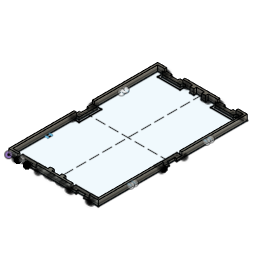
eNSPanel v2.1.4 enclosure (Autodesk Fusion 360 design; units mm, degrees)
Autodesk Fusion 360 part; units mm, degrees
note: some values were not read from the file. Chosen so that the rebuilt part matches the saved one: which bodies a step acts on; which face or edge a step refers to.
sketch "Sketch1" plane through (0, 0, 0) normal (0, 0, 1) x (1, 0, 0)
  line L0 (21, 0) -> (21, 3.8)
  line L1 (21, 3.8) -> (7, 3.8)
  line L2 (7, 3.8) -> (7, 0)
  line L3 (17, 0) -> (17, 1.4)
  line L4 (17, 1.4) -> (11, 1.4)
  line L5 (11, 1.4) -> (11, 0)
  line L6 (0, 57.2) -> (68.8, 57.2) construction
  line L7 (34.4, 114.4) -> (34.4, 0) construction
  line L8 (47.8, 0) -> (47.8, 3.8)
  line L9 (47.8, 3.8) -> (61.8, 3.8)
  line L10 (61.8, 3.8) -> (61.8, 0)
  line L11 (51.8, 1.4) -> (57.8, 1.4)
  line L12 (57.8, 1.4) -> (57.8, 0)
  line L13 (51.8, 0) -> (51.8, 1.4)
  line L14 (7, 110.6) -> (7, 114.4)
  line L15 (21, 110.6) -> (7, 110.6)
  line L16 (21, 114.4) -> (21, 110.6)
  line L17 (17, 113) -> (11, 113)
  line L18 (11, 113) -> (11, 114.4)
  line L19 (17, 114.4) -> (17, 113)
  line L20 (47.8, 114.4) -> (47.8, 110.6)
  line L21 (47.8, 110.6) -> (61.8, 110.6)
  line L22 (51.8, 113) -> (57.8, 113)
  line L23 (51.8, 114.4) -> (51.8, 113)
  line L24 (57.8, 113) -> (57.8, 114.4)
  line L25 (61.8, 110.6) -> (61.8, 114.4)
  line L26 (68.8, 54.2) -> (67.4, 54.2)
  line L27 (67.4, 54.2) -> (67.4, 60.2)
  line L28 (67.4, 60.2) -> (68.8, 60.2)
  line L29 (68.8, 50.2) -> (65, 50.2)
  line L30 (65, 50.2) -> (65, 64.2)
  line L31 (65, 64.2) -> (68.8, 64.2)
  line L32 (3.8, 64.2) -> (0, 64.2)
  line L33 (3.8, 50.2) -> (3.8, 64.2)
  line L34 (0, 50.2) -> (3.8, 50.2)
  line L35 (0, 54.2) -> (1.4, 54.2)
  line L36 (1.4, 54.2) -> (1.4, 60.2)
  line L37 (1.4, 60.2) -> (0, 60.2)
  line L38 (7, 0) -> (11, 0)
  line L39 (17, 0) -> (21, 0)
  line L40 (0, 0) -> (11, 0)
  line L41 (17, 0) -> (51.8, 0)
  line L42 (57.8, 0) -> (68.8, 0)
  line L43 (68.8, 0) -> (68.8, 54.2)
  line L44 (68.8, 60.2) -> (68.8, 114.4)
  line L45 (68.8, 64.2) -> (68.8, 60.2)
  line L46 (68.8, 54.2) -> (68.8, 50.2)
  line L47 (0, 114.4) -> (0, 60.2)
  line L48 (0, 54.2) -> (0, 0)
  line L49 (11, 114.4) -> (0, 114.4)
  line L50 (68.8, 114.4) -> (57.8, 114.4)
  line L51 (51.8, 114.4) -> (17, 114.4)
  line L52 (18.6, 1.6) -> (50.2, 1.6)
  line L53 (50.2, 1.6) -> (50.2, 3)
  line L54 (50.2, 3) -> (59.4, 3)
  line L55 (59.4, 3) -> (59.4, 1.6)
  line L56 (59.4, 1.6) -> (67.2, 1.6)
  line L57 (67.2, 1.6) -> (67.2, 52.6)
  line L58 (67.2, 52.6) -> (65.8, 52.6)
  line L59 (65.8, 52.6) -> (65.8, 61.8)
  line L60 (65.8, 61.8) -> (67.2, 61.8)
  line L61 (67.2, 61.8) -> (67.2, 112.8)
  line L62 (67.2, 112.8) -> (59.4, 112.8)
  line L63 (18.6, 1.6) -> (18.6, 3)
  line L64 (18.6, 3) -> (9.4, 3)
  line L65 (9.4, 3) -> (9.4, 1.6)
  line L66 (8.5, 1.6) -> (9.4, 1.6)
  line L67 (1.6, 52.6) -> (1.6, 1.6)
  line L68 (1.6, 1.6) -> (9.4, 1.6)
  line L69 (1.6, 52.6) -> (3, 52.6)
  line L70 (3, 52.6) -> (3, 61.8)
  line L71 (3, 61.8) -> (1.6, 61.8)
  line L72 (1.6, 112.8) -> (1.6, 61.8)
  line L73 (67.2, 112.8) -> (59.4, 112.8)
  line L74 (59.4, 111.4) -> (59.4, 112.8)
  line L75 (50.2, 111.4) -> (59.4, 111.4)
  line L76 (50.2, 112.8) -> (50.2, 111.4)
  line L77 (50.2, 112.8) -> (18.6, 112.8)
  line L78 (18.6, 112.8) -> (18.6, 111.4)
  line L79 (18.6, 111.4) -> (9.4, 111.4)
  line L80 (9.4, 111.4) -> (9.4, 112.8)
  line L81 (9.4, 112.8) -> (1.6, 112.8)
  line L82 (22.6, 114.4) -> (22.6, 109)
  line L83 (22.6, 109) -> (5.4, 109)
  line L84 (5.4, 109) -> (5.4, 114.4)
  line L85 (46.2, 114.4) -> (46.2, 109)
  line L86 (46.2, 109) -> (63.4, 109)
  line L87 (63.4, 109) -> (63.4, 114.4)
  line L88 (68.8, 48.6) -> (63.4, 48.6)
  line L89 (63.4, 48.6) -> (63.4, 65.8)
  line L90 (63.4, 65.8) -> (68.8, 65.8)
  line L91 (46.2, 0) -> (46.2, 5.4)
  line L92 (46.2, 5.4) -> (63.4, 5.4)
  line L93 (63.4, 5.4) -> (63.4, 0)
  line L94 (22.6, 0) -> (22.6, 5.4)
  line L95 (22.6, 5.4) -> (5.4, 5.4)
  line L96 (5.4, 5.4) -> (5.4, 0)
  line L97 (0, 48.6) -> (5.4, 48.6)
  line L98 (5.4, 48.6) -> (5.4, 65.8)
  line L99 (5.4, 65.8) -> (0, 65.8)
  line L100 (1.6, 29.4948) -> (3.6, 29.4948)
  line L101 (3.6, 29.4948) -> (3.6, 26.4948)
  line L102 (3.6, 26.4948) -> (1.6, 26.4948)
  line L103 (1.6, 26.4948) -> (1.6, 29.4948)
  line L104 (67.2, 29.4948) -> (65.2, 29.4948)
  line L105 (65.2, 29.4948) -> (65.2, 26.4948)
  line L106 (65.2, 26.4948) -> (67.2, 26.4948)
  line L107 (67.2, 84.9052) -> (65.2, 84.9052)
  line L108 (65.2, 84.9052) -> (65.2, 87.9052)
  line L109 (65.2, 87.9052) -> (67.2, 87.9052)
  line L110 (3.6, 84.9052) -> (3.6, 87.9052)
  line L111 (1.6, 84.9052) -> (3.6, 84.9052)
  line L112 (3.6, 87.9052) -> (1.6, 87.9052)
  line L113 (28.4, 112.8) -> (31.4, 112.8)
  line L114 (31.4, 112.8) -> (31.4, 110.8)
  line L115 (31.4, 110.8) -> (28.4, 110.8)
  line L116 (28.4, 110.8) -> (28.4, 112.8)
  line L117 (28.4, 3.6) -> (28.4, 1.6)
  line L118 (31.4, 3.6) -> (28.4, 3.6)
  line L119 (31.4, 1.6) -> (31.4, 3.6)
  line L120 (37.4, 110.8) -> (40.4, 110.8)
  line L121 (40.4, 110.8) -> (40.4, 112.8)
  line L122 (37.4, 112.8) -> (37.4, 110.8)
  line L123 (37.4, 1.6) -> (37.4, 3.6)
  line L124 (37.4, 3.6) -> (40.4, 3.6)
  line L125 (40.4, 3.6) -> (40.4, 1.6)
  point P0 (14, 0)
  point P1 (14, 0)
  point P2 (7, 0)
  point P3 (14, 0)
  point P4 (68.8, 50.2)
  dimension "d10" = 68.8
  dimension "d11" = 114.4
  dimension "d12" = 14
  dimension "d13" = 7
  dimension "d14" = 3
  dimension "d15" = 14
  dimension "d16" = 3.8
  dimension "d17" = 6
  dimension "d18" = 1.4
  dimension "d19" = 3
  dimension "d20" = 7
  dimension "d21" = 1.4
  dimension "d22" = 6
  dimension "d23" = 3.8
  dimension "d24" = 14
  dimension "d30" = -1.6
  dimension "d31" = 1.6
  dimension "d32" = -1.6
  dimension "d33" = -1.6
  dimension "d34" = 1.6
  dimension "d35" = 1.6
  dimension "d36" = 2
  dimension "d37" = 3
  dimension "d38" = 3
  dimension "d39" = 2
  dimension "d40" = 6
  constraint horizontal L40
  constraint vertical L43
  constraint horizontal L50
  constraint vertical L47
  constraint coincident L40.start L48.end
  constraint coincident P3 L40
  constraint coincident P3 P1
  constraint coincident P2 L40
  constraint horizontal L38
  constraint vertical L0
  constraint horizontal L1
  constraint vertical L2
  constraint coincident P2 L2.end
  constraint vertical L3
  constraint horizontal L4
  constraint vertical L5
  constraint coincident L5.end L38.end
  constraint symmetric P2 L7 L10.end
  constraint symmetric L0.start L7 L8.start
  constraint symmetric L0.end L7 L8.end
  constraint symmetric L1.end L7 L9.end
  constraint symmetric L5.end L7 L12.end
  constraint symmetric L3.start L7 L13.start
  constraint symmetric L3.end L7 L11.start
  constraint symmetric L4.end L7 L11.end
  constraint symmetric P2 L6 L14.end
  constraint symmetric L0.start L6 L16.start
  constraint symmetric L0.end L6 L15.start
  constraint symmetric L1.end L6 L14.start
  constraint symmetric L5.end L6 L18.end
  constraint symmetric L3.start L6 L19.start
  constraint symmetric L3.end L6 L17.start
  constraint symmetric L4.end L6 L17.end
  constraint symmetric L6 L8.start L20.start
  constraint symmetric L6 L8.end L20.end
  constraint symmetric L6 L9.end L21.end
  constraint symmetric L6 L10.end L25.end
  constraint symmetric L6 L11.start L22.start
  constraint symmetric L6 L11.end L22.end
  constraint symmetric L6 L12.end L24.end
  constraint symmetric L6 L13.start L23.start
  constraint coincident P4 L43
  constraint horizontal L26
  constraint vertical L27
  constraint horizontal L28
  constraint coincident L26.start L43.end
  constraint horizontal L29
  constraint vertical L30
  constraint horizontal L31
  constraint vertical L45
  constraint coincident P4 L29.start
  constraint symmetric L7 L26.start L35.start
  constraint symmetric L7 L26.end L35.end
  constraint symmetric L7 L27.end L36.end
  constraint symmetric L7 L28.end L37.end
  constraint symmetric L7 P4 L34.start
  constraint symmetric L7 L29.end L33.start
  constraint symmetric L7 L30.end L32.start
  constraint symmetric L7 L31.end L32.end
  constraint collinear L38 L39
  constraint collinear L40 L41
  constraint coincident L7.end L40
  constraint collinear L41 L42
  constraint collinear L43 L44
  constraint coincident L6.end L43
  constraint collinear L45 L46
  constraint collinear L47 L48
  constraint coincident L6.start L47
  constraint collinear L49 L50
  constraint coincident L7.start L50
  constraint collinear L50 L51
  constraint horizontal L100
  constraint vertical L101
  constraint horizontal L102
  constraint vertical L103
  constraint coincident L67 L100.start
  constraint symmetric L7 L100.start L104.start
  constraint symmetric L7 L100.end L104.end
  constraint symmetric L7 L101.end L105.end
  constraint symmetric L7 L102.end L106.end
  constraint symmetric L6 L100.start L111.start
  constraint symmetric L6 L100.end L110.start
  constraint symmetric L6 L101.end L110.end
  constraint symmetric L6 L102.end L112.end
  constraint symmetric L6 L104.start L107.start
  constraint symmetric L6 L104.end L107.end
  constraint symmetric L6 L105.end L108.end
  constraint symmetric L6 L106.end L109.end
  constraint horizontal L113
  constraint vertical L114
  constraint horizontal L115
  constraint vertical L116
  constraint coincident L77 L113.start
  constraint symmetric L6 L113.start L117.end
  constraint symmetric L6 L113.end L119.start
  constraint symmetric L6 L114.end L118.start
  constraint symmetric L6 L115.end L117.start
  constraint symmetric L7 L113.start L121.end
  constraint symmetric L7 L113.end L122.start
  constraint symmetric L7 L114.end L120.start
  constraint symmetric L7 L115.end L120.end
  constraint symmetric L6 L120.start L123.end
  constraint symmetric L6 L120.end L124.end
  constraint symmetric L6 L121.end L125.end
  constraint symmetric L6 L122.start L123.start
  measures "d10" distance of L40.start L42.end
  measures "d11" distance of L40.start L47.start
  measures "d12" distance of L40.start P3
  measures "d13" distance of P3 P2
  measures "d14" distance of P3 L5.end
  measures "d15" distance of P2 L0.start
  measures "d16" distance of P2 L1.end
  measures "d17" distance of L5.end L3.start
  measures "d18" distance of L5.end L4.end
  measures "d19" distance of L6.end L26.start
  measures "d20" distance of L6.end P4
  measures "d21" distance of L26.start L26.end
  measures "d22" distance of L26.start L28.end
  measures "d23" distance of P4 L29.end
  measures "d24" distance of P4 L31.end
  measures "d36" distance of L100.start L100.end
  measures "d37" distance of L100.start L102.end
  measures "d38" distance of L113.start L113.end
  measures "d39" distance of L113.start L115.end
  measures "d40" distance of L7 L113.start
extrude "Extrude1" add sketch "Sketch1" along normal blind 4.2 contours L0 L41 L52 L94 | L41 L52 L91 L94 | L8 L41 L52 L91 | L52 L117 L118 L119 | L2 L40 L68 L96 | L52 L123 L124 L125 | L40 L48 L67 L68 L96 L97 L103 | L10 L42 L56 L93 | L42 L43 L56 L57 L88 L93 | L34 L48 L67 L97 | L29 L43 L57 L88 | L47 L49 L72 L81 L84 L99 | L32 L47 L72 L99 | L31 L44 L61 L90 | L44 L50 L61 L62 L73 L87 L90 | L14 L49 L81 L84 | L25 L50 L62 L73 L87 | L51 L77 L82 L85 L113 | L16 L51 L77 L82 | L77 L113 L114 L115 L116 | L20 L51 L77 L85 | L77 L120 L121 L122 makes body 1 at (0, 97.6667, 1.4) makes body 2 at (68.8, 16.7333, 2.8) makes body 3 at (0, 33.4667, 2.8) makes body 4 at (38.8667, 114.4, 1.4) makes body 5 at (68.8, 80.9333, 1.4) makes body 6 at (29.9333, 0, 2.8)
extrude "Extrude2" add sketch "Sketch1" along normal blind 1.8 contours L0 L2 L3 L4 L5 L38 L39 L40 L41 L52 L63 L64 L65 L66 L68 | L0 L1 L2 L52 L63 L64 L65 L66 L68 | L8 L10 L11 L12 L13 L41 L42 L52 L53 L54 L55 L56 | L8 L9 L10 L52 L53 L54 L55 L56 | L32 L34 L35 L36 L37 L47 L48 L67 L69 L70 L71 L72 | L32 L33 L34 L67 L69 L70 L71 L72 | L26 L27 L28 L29 L31 L43 L44 L45 L46 L57 L58 L59 L60 L61 | L29 L30 L31 L57 L58 L59 L60 L61 | L14 L16 L17 L18 L19 L49 L51 L77 L78 L79 L80 L81 | L14 L15 L16 L77 L78 L79 L80 L81 | L20 L22 L23 L24 L25 L50 L51 L62 L73 L74 L75 L76 L77 | L20 L21 L25 L62 L73 L74 L75 L76 L77 bodies 1 5 2 4 3 6
fillet "Fillet1" radius 2 8 edges at (7, 112.8, 0.9) (21, 112.8, 0.9) (47.8, 112.8, 0.9) (7, 1.6, 0.9) (61.8, 112.8, 0.9) (21, 1.6, 0.9) (47.8, 1.6, 0.9) (61.8, 1.6, 0.9) on bodies 1
ref_plane "WorkPlane1" through (0, 57.2, 0) normal (0, 1, 0) x (0, 0, 1)
equation "width = 68.8 mm"
equation "height = 114.4 mm"
equation "depth = 4.2 mm"
equation "inner_depth = 1.6 mm"
equation "insets_width = 14 mm"
equation "insets_height = 3.8 mm"
equation "insets_niche_depth = 1.4 mm"
equation "insets_niche_width = 6 mm"
equation "insets_topbot_center_from_edge = 14 mm"
equation "d10 = width"
equation "d11 = height"
equation "d12 = insets_topbot_center_from_edge"
equation "d13 = insets_width / 2"
equation "d14 = insets_niche_width / 2"
equation "d15 = insets_width"
equation "d16 = insets_height"
equation "d17 = insets_niche_width"
equation "d18 = insets_niche_depth"
equation "d19 = insets_niche_width / 2"
equation "d20 = insets_width / 2"
equation "d21 = insets_niche_depth"
equation "d22 = insets_niche_width"
equation "d23 = insets_height"
equation "d24 = insets_width"
equation "d41 = depth"
equation "d49 = height / 2"
